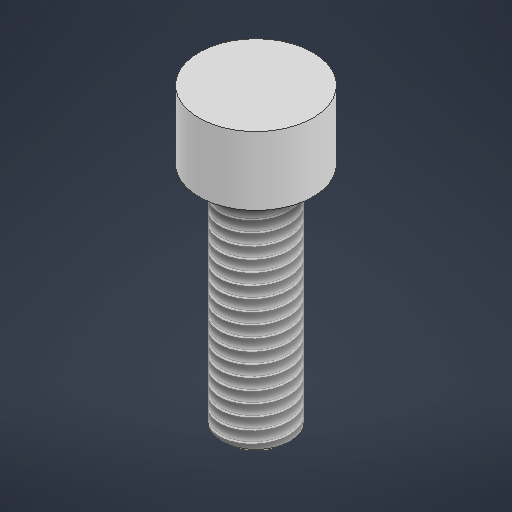
# Autodesk Inventor part: 01-03-01-02 Schraube kl.
Saved by Autodesk Inventor 2026.2 (Build 302298000, 298)
## iProperties
Created: 2026-01-31
Part Number: 01-03-01-02 Schraube kl.
Material: Generisch
Document SubType Name: Modeling
Designer: Schally
Density: 1 g/cm^3
Appearance: Vorgabe
Author: Schally
Autodesk Inventor part; units mm, degrees
ref_plane "YZ Plane" through (0, 0, 0) normal (1, 0, 0) x (0, 1, 0)
ref_plane "XZ Plane" through (0, 0, 0) normal (0, 1, 0) x (-1, 0, 0)
ref_plane "XY Plane" through (0, 0, 0) normal (0, 0, 1) x (1, 0, 0)
sketch "Skizze1" plane through (0, 0, 0) normal (1, 0, 0) x (0, 1, 0)
  line L0 (-2.6, 0) -> (15.6, 0) projected
  line L1 (0, -3) -> (0, 0.5) projected
  line L2 (0, 0) -> (0, -1.5)
  line L3 (0, -1.5) -> (10, -1.5)
  line L4 (10, -1.5) -> (10, -2.5)
  line L5 (10, -2.5) -> (13, -2.5)
  line L6 (13, -2.5) -> (13, 0)
  dimension "d0" = 1.5
  dimension "d1" = 10
  dimension "d2" = 1
  dimension "d3" = 3
  constraints: 10 end point, 3 perpendicular, 2 point on line, 1 parallel
  measures "d0" distance of L2.start L2.end
  measures "d1" distance of L2.end L3.end
  measures "d2" distance of L3.end L4.end
  measures "d3" distance of L4.end L5.end
revolve "Umdrehung1" add sketch "Skizze1" angle 360 about axis through (0, -10, 0) along (0, 1, 0)
thread "Gewinde1" size "M3x0.5" class "6g" standard "ANSI Metric M Profile" length 24
chamfer "Fasen1" distance 0.2 angle 45 1 edges at (0, 0, 1.5)
